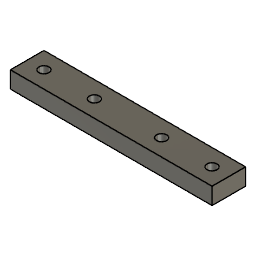
Probeta_Experimento_4_Puntas (Autodesk Fusion 360 design; units mm, degrees)
part number: 2025-12-05-10-06-00-199
Autodesk Fusion 360 part; units mm, degrees
sketch "Boceto1" plane through (0, 0, 0) normal (0, 0, 1) x (1, 0, 0)
  line L0 (30, 5) -> (-30, 5)
  line L1 (-30, 5) -> (-30, -5)
  line L2 (-30, -5) -> (30, -5)
  line L3 (30, -5) -> (30, 5)
  line L4 (30, 5) -> (-30, -5) construction
  line L5 (-30, 5) -> (30, -5) construction
  dimension "d1" = 60
  dimension "d2" = 10
  constraint horizontal L0
  constraint perpendicular L0 L1
  constraint parallel L0 L2
  constraint parallel L1 L3
  constraint coincident L4 origin
  constraint coincident L5 origin
  measures "d1" distance of L1.end L2.end
  measures "d2" distance of L0.end L1.end
extrude "Extruir1" add sketch "Boceto1" along normal blind 5
hole "Agujero1" at (25, 0, 5) direction (0, 0, -1) diameter 3 depth 8 tip angle 180
hole "Agujero2" at (-25, 0, 5) direction (0, 0, -1) diameter 3 depth 8 tip angle 180
hole "Agujero3" at (-10, 0, 5) direction (0, 0, -1) diameter 3 depth 3 tip angle 180
hole "Agujero4" at (10, 0, 5) direction (0, 0, -1) diameter 3 depth 3 tip angle 180
move_body "Desplazar3" bodies 1 to x (1, 0, 0) y (0, 1, 0) z (0, 0, 1) at (0, 27, 0)
